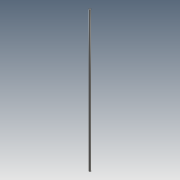
# Autodesk Inventor part: eixo-cromado-16h7
Saved by Autodesk Inventor 2017 (Build 210142000, 142)
## iProperties
Created: 2018-05-19
Part Number: eixo-cromado-16h7
Material: Stainless Steel
Document SubType Name: Modeling
Designer: Luiz Gustavo
Density: 8 g/cm^3
Appearance: Steel - Polished
Author: Luiz Gustavo
Autodesk Inventor part; units mm, degrees
ref_plane "YZ Plane" through (0, 0, 0) normal (1, 0, 0) x (0, 1, 0)
ref_plane "XZ Plane" through (0, 0, 0) normal (0, 1, 0) x (-1, 0, 0)
ref_plane "XY Plane" through (0, 0, 0) normal (0, 0, 1) x (1, 0, 0)
sketch "Sketch1" plane through (0, 0, 0) normal (0, 1, 0) x (-1, 0, 0)
  line L0 (0, -657.5) -> (0, 657.5)
  line L1 (0, -657.5) -> (8, -657.5)
  line L2 (8, -657.5) -> (8, 657.5)
  line L3 (8, 657.5) -> (0, 657.5)
  point P0 (0, 0)
  point P1 (0, 0)
  dimension "d0" = 1315
  dimension "d3" = 16
  constraints: 8 end point, 2 perpendicular, 1 coincident, 1 horizontal, 1 midpoint, 1 vertical
  measures "d0" distance of L0.start L0.end
  measures "d3" diameter of L2 L0
revolve "Revolution1" add sketch "Sketch1" angle 360 about axis through (0, 0, -657.5) along (0, 0, 1)
body "Solid1"
